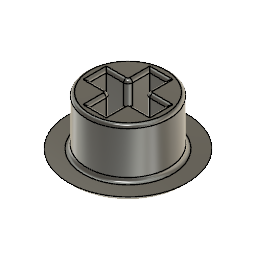
Assembly10Tilt7 v4 (Autodesk Fusion 360 archive; units mm, degrees)
design "MX Plug Mushroom"
Autodesk Fusion 360 part; units mm, degrees
sketch "Sketch1" plane through (0, 0, 0) normal (0, 0, 1) x (1, 0, 0)
  circle A0 centre (0, 0) radius 2.75
  line L0 (0.585, -2.05) -> (-0.585, -2.05)
  line L1 (-0.585, 0.885) -> (-0.585, 2.05)
  line L2 (-0.585, 2.05) -> (0.585, 2.05)
  line L3 (0.585, -0.885) -> (0.585, -2.05)
  line L4 (0.585, -2.05) -> (-0.585, 2.05) construction
  line L5 (-0.585, -2.05) -> (0.585, 2.05) construction
  line L6 (2.05, -0.585) -> (0.885, -0.585)
  line L7 (-2.05, -0.585) -> (-2.05, 0.585)
  line L8 (0.885, 0.585) -> (2.05, 0.585)
  line L9 (2.05, 0.585) -> (2.05, -0.585)
  line L10 (2.05, -0.585) -> (-2.05, 0.585) construction
  line L11 (-2.05, -0.585) -> (2.05, 0.585) construction
  arc A1 (0.885, -0.585) -> (0.585, -0.885) centre (0.885, -0.885) ccw
  line L12 (0.585, 2.05) -> (0.585, 0.885)
  arc A2 (0.585, 0.885) -> (0.885, 0.585) centre (0.885, 0.885) ccw
  line L13 (-2.05, 0.585) -> (-0.885, 0.585)
  line L14 (-2.05, -0.585) -> (-0.885, -0.585)
  arc A3 (-0.885, 0.585) -> (-0.585, 0.885) centre (-0.885, 0.885) ccw
  line L15 (-0.585, -0.885) -> (-0.585, -2.05)
  arc A4 (-0.585, -0.885) -> (-0.885, -0.585) centre (-0.885, -0.885) ccw
  point P0 (0.585, -0.585)
  dimension "d1" = 5.5
  dimension "d2" = 1.17
  dimension "d3" = 4.1
  dimension "d4" = 4.1
  dimension "d5" = 1.17
  dimension "d6" = 0.3
  dimension "d7" = 0.3
  dimension "d8" = 0.3
  dimension "d9" = 0.3
  constraint coincident A0.centre origin
  constraint horizontal L0
  constraint perpendicular L0 L1
  constraint parallel L0 L2
  constraint parallel L1 L3
  constraint coincident L4 A0.centre
  constraint coincident L5 A0.centre
  constraint horizontal L6
  constraint perpendicular L6 L7
  constraint parallel L6 L8
  constraint parallel L7 L9
  constraint coincident L10 A0.centre
  constraint coincident L11 A0.centre
  constraint coincident L3 P0
  constraint coincident L6 P0
  constraint coincident L7.start L6
  constraint coincident L2.end L3
  constraint tangent L6 A1
  constraint tangent L3 A1
  constraint perpendicular L8 L12
  constraint coincident L7.end L8
  constraint tangent L8 A2
  constraint tangent L12 A2
  constraint perpendicular L1 L13
  constraint perpendicular L1 L14
  constraint coincident L0.end L1
  constraint tangent L13 A3
  constraint tangent L1 A3
  constraint tangent L15 A4
  constraint tangent L14 A4
  constraint parallel L3 L15
  measures "d1" diameter of A0
  measures "d2" distance of L1.end L2.end
  measures "d3" distance of L0.start L2.end
  measures "d4" distance of L7.end L8.end
  measures "d5" distance of L7.start L7.end
  measures "d6" radius of A1
  measures "d7" radius of A2
  measures "d8" radius of A3
  measures "d9" radius of A4
extrude "Extrude1" add sketch "Sketch1" along normal blind 3.3
sketch "Sketch2" plane through (0, 0, 0) normal (0, 0, -1) x (1, 0, 0)
  line L0 (-2.05, 0.585) -> (-0.885, 0.585)
  arc A0 (-0.885, 0.585) -> (-0.585, 0.885) centre (-0.885, 0.885) ccw
  line L1 (-0.585, 0.885) -> (-0.585, 2.05)
  line L2 (-0.585, 2.05) -> (0.585, 2.05)
  line L3 (0.585, 2.05) -> (0.585, 0.885)
  arc A1 (0.585, 0.885) -> (0.885, 0.585) centre (0.885, 0.885) ccw
  line L4 (0.885, 0.585) -> (2.05, 0.585)
  line L5 (2.05, 0.585) -> (2.05, -0.585)
  line L6 (2.05, -0.585) -> (0.885, -0.585)
  arc A2 (0.885, -0.585) -> (0.585, -0.885) centre (0.885, -0.885) ccw
  line L7 (0.585, -0.885) -> (0.585, -2.05)
  line L8 (0.585, -2.05) -> (-0.585, -2.05)
  line L9 (-0.585, -2.05) -> (-0.585, -0.885)
  arc A3 (-0.585, -0.885) -> (-0.885, -0.585) centre (-0.885, -0.885) ccw
  line L10 (-0.885, -0.585) -> (-2.05, -0.585)
  line L11 (-2.05, -0.585) -> (-2.05, 0.585)
  circle A4 centre (0, 0) radius 2.75
  line L12 (4, 4) -> (-4, 4)
  line L13 (-4, 4) -> (-4, -4)
  line L14 (-4, -4) -> (4, -4)
  line L15 (4, -4) -> (4, 4)
  line L16 (4, 4) -> (-4, -4) construction
  line L17 (-4, 4) -> (4, -4) construction
  dimension "d12" = 8
  dimension "d13" = 8
  constraint horizontal L12
  constraint perpendicular L12 L13
  constraint parallel L12 L14
  constraint parallel L13 L15
  constraint coincident L16 A4.centre
  constraint coincident L17 A4.centre
  constraint coincident A4.centre origin
  measures "d12" distance of L13.end L14.end
  measures "d13" distance of L12.end L13.end
extrude "Extrude2" add sketch "Sketch2" along normal blind 0.94 contours L0 A0 L1 L2 L3 A1 L4 L5 L6 A2 L7 L8 L9 A3 L10 L11 | A4 | L12 L13 L14 L15
fillet "Fillet1" radius 0.25 1 edges at (-2.5639, -0.9944, 0)
fillet "Fillet2" radius 0.2 1 edges at (-2.5639, -0.9944, 3.3)
fillet "Fillet3" radius 0.2 16 edges at (1.4675, -0.585, 3.3) (0.6729, -0.6729, 3.3) (0.585, -1.4675, 3.3) (2.05, 0, 3.3) (0.585, 1.4675, 3.3) (0.6729, 0.6729, 3.3) (1.4675, 0.585, 3.3) (0, 2.05, 3.3) (-1.4675, 0.585, 3.3) (-0.6729, 0.6729, 3.3) (-0.585, 1.4675, 3.3) (-2.05, 0, 3.3) (-0.585, -1.4675, 3.3) (-0.6729, -0.6729, 3.3) (-1.4675, -0.585, 3.3) (0, -2.05, 3.3)
ref_plane "WorkPlane1" through (0, 0, 0) normal (1, 0, 0) x (0, 1, 0)
sketch "Sketch6" plane through (0, 0, 0) normal (1, 0, 0) x (0, 1, 0)
  line L0 (4, 0) -> (-4, 0)
  line L1 (-4, 0) -> (-4, -0.94)
  line L2 (-4, -0.94) -> (4, -0.94)
  line L3 (4, -0.94) -> (4, 0)
  line L4 (0, 2.5) -> (0, -1.5)
  constraint vertical L4
sketch "Sketch3" plane through (0, 0, 0) normal (1, 0, 0) x (0, 1, 0)
  spline S0 degree 5 poles (4, 0) (3.9112, -0.1331) (3.7126, -0.3686) (3.3515, -0.6292) (2.7612, -0.8192) (1.9044, -0.8968) (1.1633, -0.9019) (0.5883, -0.9003) (0.1974, -0.9) (0, -0.9) knots 0 0 0 0 0 0 0.2 0.4 0.6 0.8 1 1 1 1 1 1
  line L0 (4.2, 0.3) -> (3.8, -0.3)
  line L1 (0.5, -0.9) -> (-0.5, -0.9)
  line L2 (4, 0) -> (4, -1)
  line L3 (4, -1) -> (0, -1)
  line L4 (0, -1) -> (0, -0.9)
  line L5 (4, 0) -> (7, 0)
  line L6 (7, 0) -> (7, -1)
  line L7 (7, -1) -> (4, -1)
  line L8 (4, -1) -> (4, 0)
  constraint midpoint S0.start L0
  constraint midpoint L1 S0.end
  constraint vertical L2
  constraint perpendicular L2 L3
  constraint perpendicular L3 L4
  constraint horizontal L5
  constraint vertical L6
  constraint horizontal L7
  constraint vertical L8
sketch "Sketch4" plane through (0, -4, 0) normal (0, -1, 0) x (1, 0, 0)
  line L0 (4, 0) -> (-4, 0)
  constraint horizontal L0
revolve "Revolve1" cut sketch "Sketch3" angle 360 about axis through (0, 0, 2.5) along (0, 0, -1)
sweep "Sweep1" [suppressed]
